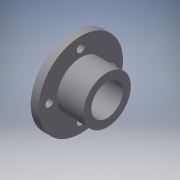
# Autodesk Inventor part: Flange
Saved by Autodesk Inventor 2019 (Build 230136000, 136)
## iProperties
Created: 2019-01-14
Part Number: Flange
Material: Generic
Document SubType Name: Modeling
Designer: nxgam
Density: 1 g/cm^3
Appearance: Default
Author: nxgam
Autodesk Inventor part; units mm, degrees
ref_plane "YZ Plane" through (0, 0, 0) normal (1, 0, 0) x (0, 1, 0)
ref_plane "XZ Plane" through (0, 0, 0) normal (0, 1, 0) x (-1, 0, 0)
ref_plane "XY Plane" through (0, 0, 0) normal (0, 0, 1) x (1, 0, 0)
sketch "Sketch1" plane through (0, 0, 0) normal (1, 0, 0) x (0, 1, 0)
  circle A0 centre (0, 0) radius 16
  dimension "d0" = 32
  constraints: 1 centre point, 1 coincident
  measures "d0" diameter of A0
extrude "Extrusion1" add sketch "Sketch1" along normal blind 3
sketch "Sketch2" plane through (3, 0, 0) normal (1, 0, 0) x (0, 0, -1)
  circle A0 centre (0, 0) radius 9
  dimension "d3" = 18
  constraints: 1 centre point, 1 coincident
  measures "d3" diameter of A0
extrude "Extrusion2" add sketch "Sketch2" along normal blind 10
sketch "Sketch3" plane through (13, 0, 0) normal (1, 0, 0) x (0, 0, -1)
  circle A0 centre (0, 0) radius 6
  dimension "d6" = 12
  constraints: 1 centre point, 1 coincident
  measures "d6" diameter of A0
extrude "Extrusion3" cut sketch "Sketch3" against normal through all
sketch "Sketch4" plane through (3, 0, 0) normal (1, 0, 0) x (0, 0, -1)
  circle A0 centre (0, 0) radius 9 projected
  circle A1 centre (0, 0) radius 16 projected
  point P0 (0, 11.938)
  point P1 (-11.938, 0)
  point P2 (0, -11.938)
  point P3 (11.938, 0)
  dimension "d9" = 11.938
  dimension "d10" = 32
  dimension "d11" = 18
  dimension "d14" = 360
  constraints: 5 other
  measures "d9" distance of point (0, 11.938) point (0, 0)
  measures "d10" diameter of A1
  measures "d11" diameter of A0
hole "Hole1" at (3, 11.938, 0) at (3, 0, 11.938) at (3, -11.938, 0) at (3, 0, -11.938) direction (-1, 0, 0) diameter 3 end through all
body "Solid1"
